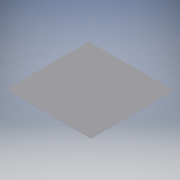
# Autodesk Inventor part: Part29
Saved by Autodesk Inventor 2018 (Build 220112000, 112)
## iProperties
Created: 2019-05-29
Part Number: Part29
Material: Generic
Document SubType Name: Modeling
Designer: Ash
Density: 1 g/cm^3
Appearance: Default
Author: Ash
Autodesk Inventor part; units mm, degrees
ref_plane "YZ Plane" through (0, 0, 0) normal (1, 0, 0) x (0, 1, 0)
ref_plane "XZ Plane" through (0, 0, 0) normal (0, 1, 0) x (-1, 0, 0)
ref_plane "XY Plane" through (0, 0, 0) normal (0, 0, 1) x (1, 0, 0)
sketch "Sketch1" plane through (0, 0, 0) normal (0, 1, 0) x (-1, 0, 0)
  line L0 (0, 0) -> (48.271, 0)
  line L1 (48.271, 0) -> (48.271, -47.0385)
  line L2 (48.271, -47.0385) -> (0, -47.0385)
  line L3 (0, -47.0385) -> (0, 0)
  constraints: 8 end point, 2 parallel, 1 horizontal, 1 perpendicular
extrude "Extrusion1" add sketch "Sketch1" along normal blind 0.0254
body "Solid1"
